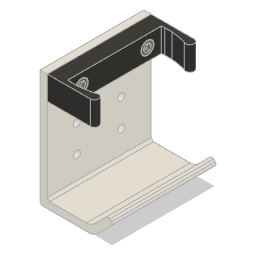
Zippo carry v8 (Autodesk Fusion 360 design; units mm, degrees)
Autodesk Fusion 360 part; units mm, degrees
note: some values were not read from the file. Chosen so that the rebuilt part matches the saved one: which bodies a step acts on. Set by a fixed rule: which sketch regions a step uses.
sketch "Sketch1" plane through (0, 0, 0) normal (1, 0, 0) x (0, 0, -1)
  line L0 (19.25, 28.375) -> (-19.25, 28.375)
  line L1 (-19.25, 28.375) -> (-19.25, -28.375)
  line L2 (-19.25, -28.375) -> (19.25, -28.375)
  line L3 (19.25, -28.375) -> (19.25, 28.375)
  line L4 (19.25, 28.375) -> (-19.25, -28.375) construction
  line L5 (-19.25, 28.375) -> (19.25, -28.375) construction
  dimension "d1" = 38.5
  dimension "d2" = 56.75
  constraint horizontal L0
  constraint perpendicular L0 L1
  constraint parallel L0 L2
  constraint parallel L1 L3
  constraint coincident L4 origin
  constraint coincident L5 origin
  measures "d1" distance of L1.end L2.end
  measures "d2" distance of L0.end L1.end
extrude "Extrude1" add sketch "Sketch1" along normal blind 14.75 makes body 1
sketch "Sketch2" plane through (0, 28.375, 0) normal (0, 1, 0) x (-1, 0, 0)
  line L0 (0, -19.25) -> (0, 19.25)
  line L1 (0, 19.25) -> (-14.75, 19.25)
  line L2 (-14.75, 19.25) -> (-14.75, -19.25)
  line L3 (-14.75, -19.25) -> (0, -19.25)
  line L4 (-7.375, 0) -> (-7.375, 19.3)
  line L5 (-14.75, 0) -> (-14.75, 18.2)
  line L6 (0, 0) -> (0, 18.2)
  spline S0 degree 5 poles (-14.75, 18.2) (-14.455, 18.2834) (-13.865, 18.443) (-12.98, 18.6605) (-11.8, 18.9061) (-10.325, 19.134) (-8.85, 19.2757) (-7.375, 19.3242) (-5.9, 19.2757) (-4.425, 19.134) (-2.95, 18.9061) (-1.77, 18.6605) (-0.885, 18.443) (-0.295, 18.2834) (0, 18.2) knots 0 0 0 0 0 0 0.1 0.2 0.3 0.4 0.5 0.6 0.7 0.8 0.9 1 1 1 1 1 1
  line L7 (-7.375, 0) -> (-7.375, -19.3)
  line L8 (-14.75, 0) -> (-14.75, -18.2)
  line L9 (0, 0) -> (0, -18.2)
  spline S1 degree 5 poles (-14.75, -18.2) (-14.455, -18.2834) (-13.865, -18.443) (-12.98, -18.6605) (-11.8, -18.9061) (-10.325, -19.134) (-8.85, -19.2757) (-7.375, -19.3242) (-5.9, -19.2757) (-4.425, -19.134) (-2.95, -18.9061) (-1.77, -18.6605) (-0.885, -18.443) (-0.295, -18.2834) (0, -18.2) knots 0 0 0 0 0 0 0.1 0.2 0.3 0.4 0.5 0.6 0.7 0.8 0.9 1 1 1 1 1 1
  dimension "d5" = 19.3
  dimension "d6" = 18.2
  dimension "d7" = 18.2
  dimension "d8" = 19.3
  dimension "d9" = 18.2
  dimension "d10" = 18.2
  constraint perpendicular L3 L4
  constraint midpoint L2 L5.start
  constraint parallel L2 L5
  constraint coincident L6.start L9.start
  constraint perpendicular L3 L6
  constraint parallel L4 L7
  constraint parallel L2 L8
  constraint parallel L0 L9
  measures "d5" distance of L4.start L4.end
  measures "d6" distance of L5.start L5.end
  measures "d7" distance of L6.start L6.end
  measures "d8" distance of L4.start L7.end
  measures "d9" distance of L5.start L8.end
  measures "d10" distance of L6.start L9.end
extrude "Extrude2" cut sketch "Sketch2" against normal blind 57 contours L0 L3 S1 | L3 L7 S1 | L3 L7 S1 | L0 L1 S0 | L2 L3 S1 | L1 L4 S0 | L1 L4 S0 | L1 L2 S0 bodies 1
extrude "Extrude3" add sketch "Sketch2" against normal blind 56.75 contours L3 L7 S1 | L3 L7 S1 | L1 L4 S0 | L1 L4 S0 bodies 1
ref_plane "WorkPlane1" through (-1, 0, 0) normal (-1, 0, 0) x (0, 0, 1)
sketch "Sketch3" plane through (0, 28.375, 0) normal (0, 1, 0) x (-1, 0, 0)
  spline S0 degree 5 poles (-8.887, 19.25) (-9.1746, 19.2311) (-9.7572, 19.1839) (-10.6348, 19.0861) (-11.8074, 18.9046) (-12.98, 18.6605) (-13.865, 18.443) (-14.455, 18.2834) (-14.75, 18.2) knots -0.397489 -0.397489 -0.397489 -0.397489 -0.397489 -0.397489 -0.3 -0.2 -0.1 0 0 0 0 0 0
  line L0 (-14.75, 18.2) -> (-14.75, -18.2)
  spline S1 degree 5 poles (-14.75, -18.2) (-14.455, -18.2834) (-13.865, -18.443) (-12.98, -18.6605) (-11.8074, -18.9046) (-10.6348, -19.0861) (-9.7572, -19.1839) (-9.1746, -19.2311) (-8.887, -19.25) knots 0 0 0 0 0 0 0.1 0.2 0.3 0.397489 0.397489 0.397489 0.397489 0.397489 0.397489
  spline S2 degree 5 poles (-8.887, -19.25) (-8.8796, -19.2505) (-8.5772, -19.2703) (-7.9798, -19.2997) (-7.375, -19.3099) (-6.7702, -19.2997) (-6.1728, -19.2703) (-5.8704, -19.2505) (-5.863, -19.25) knots 0.397489 0.397489 0.397489 0.397489 0.397489 0.397489 0.4 0.5 0.6 0.602511 0.602511 0.602511 0.602511 0.602511 0.602511
  spline S3 degree 5 poles (-5.863, -19.25) (-5.5754, -19.2311) (-4.9928, -19.1839) (-4.1152, -19.0861) (-2.9426, -18.9046) (-1.77, -18.6605) (-0.885, -18.443) (-0.295, -18.2834) (0, -18.2) knots 0.602511 0.602511 0.602511 0.602511 0.602511 0.602511 0.7 0.8 0.9 1 1 1 1 1 1
  line L1 (0, -18.2) -> (0, 18.2)
  spline S4 degree 5 poles (0, 18.2) (-0.295, 18.2834) (-0.885, 18.443) (-1.77, 18.6605) (-2.9426, 18.9046) (-4.1152, 19.0861) (-4.9928, 19.1839) (-5.5754, 19.2311) (-5.863, 19.25) knots -1 -1 -1 -1 -1 -1 -0.9 -0.8 -0.7 -0.602511 -0.602511 -0.602511 -0.602511 -0.602511 -0.602511
  spline S5 degree 5 poles (-8.887, 19.25) (-8.8796, 19.2505) (-8.5772, 19.2703) (-7.9798, 19.2997) (-7.375, 19.3099) (-6.7702, 19.2997) (-6.1728, 19.2703) (-5.8704, 19.2505) (-5.863, 19.25) knots 0.397489 0.397489 0.397489 0.397489 0.397489 0.397489 0.4 0.5 0.6 0.602511 0.602511 0.602511 0.602511 0.602511 0.602511
  spline S6 degree 3 poles (0.5, 18.5782) (0.3787, 18.6125) (0.2574, 18.6468) (0.1361, 18.6811) (-1.8474, 19.2421) (-3.8345, 19.6177) (-5.8302, 19.7489) knots -1.024673 -1.024673 -1.024673 -1.024673 -1 -1 -1 -0.602511 -0.602511 -0.602511 -0.602511
  spline S7 degree 3 poles (-8.9198, 19.7489) (-7.8905, 19.8166) (-6.8595, 19.8166) (-5.8302, 19.7489) knots 0.397489 0.397489 0.397489 0.397489 0.602511 0.602511 0.602511 0.602511
  spline S8 degree 3 poles (-8.9198, 19.7489) (-10.9155, 19.6177) (-12.9026, 19.2421) (-14.8861, 18.6811) (-15.0074, 18.6468) (-15.1287, 18.6125) (-15.25, 18.5782) knots -0.397489 -0.397489 -0.397489 -0.397489 0 0 0 0.024673 0.024673 0.024673 0.024673
  line L2 (-15.25, 18.5782) -> (-15.25, -18.5782)
  spline S9 degree 3 poles (-15.25, -18.5782) (-15.1287, -18.6125) (-15.0074, -18.6468) (-14.8861, -18.6811) (-12.9026, -19.2421) (-10.9155, -19.6177) (-8.9198, -19.7489) knots -0.024673 -0.024673 -0.024673 -0.024673 0 0 0 0.397489 0.397489 0.397489 0.397489
  spline S10 degree 3 poles (-8.9198, -19.7489) (-7.8905, -19.8166) (-6.8595, -19.8166) (-5.8302, -19.7489) knots 0.397489 0.397489 0.397489 0.397489 0.602511 0.602511 0.602511 0.602511
  spline S11 degree 3 poles (-5.8302, -19.7489) (-3.8345, -19.6177) (-1.8474, -19.2421) (0.1361, -18.6811) (0.2574, -18.6468) (0.3787, -18.6125) (0.5, -18.5782) knots 0.602511 0.602511 0.602511 0.602511 1 1 1 1.024673 1.024673 1.024673 1.024673
  line L3 (0.5, -18.5782) -> (0.5, 18.5782)
  line L4 (-7.375, -19.7997) -> (0.5, -19.7997)
  line L5 (0.5, -19.7997) -> (0.5, -18.5782)
  circle A0 centre (-16.125, -20.091) radius 1.7477
  line L6 (-16.125, -21.8387) -> (0.5, -21.8387)
  line L7 (0.5, -21.8387) -> (0.5, -19.7997)
  line L8 (0.5, 0) -> (-15.25, 0)
  line L9 (-16.125, 21.8387) -> (0.5, 21.8387)
  circle A1 centre (-16.125, 20.091) radius 1.7477
  line L10 (-7.375, 19.7997) -> (0.5, 19.7997)
  line L11 (0.5, 19.7997) -> (0.5, 18.5782)
  line L12 (0.5, 21.8387) -> (0.5, 19.7997)
  line L13 (0.5, -21.8387) -> (8, -21.8387)
  line L14 (8, -21.8387) -> (8, 21.8387)
  line L15 (8, 21.8387) -> (0.5, 21.8387)
  line L16 (0.5, 21.8387) -> (0.5, -21.8387)
  dimension "d16" = 0.5
  dimension "d17" = 7.5
  constraint coincident S10 L4.start
  constraint horizontal L4
  constraint perpendicular L4 L5
  constraint coincident L2.end A0
  constraint coincident A0 L6.start
  constraint tangent A0 L6
  constraint horizontal L6
  constraint midpoint L3 L8.start
  constraint midpoint L2 L8.end
  constraint perpendicular L2 L8
  constraint symmetric S11.end L8 S6.start
  constraint symmetric L4.start L8 L10.start
  constraint symmetric L4.end L8 L10.end
  constraint symmetric A0 L8 A1
  constraint symmetric L6.start L8 L9.start
  constraint symmetric L6.end L8 L9.end
  constraint horizontal L13
  constraint vertical L14
  constraint horizontal L15
  constraint vertical L16
  measures "d17" distance of L6.end L13.end
extrude "Extrude4" add sketch "Sketch3" along normal blind -2 and the other way blind 12 separate body contours L3 L5 L7 L11 L12 L13 L14 L15 L16 | S7 S8 L9 A1 L10 L12 L16 | A1 | S9 S10 L4 A0 L6 L7 L16 | A0 | S10 S11 L4 L5 L16 | S6 S7 L10 L11 L16 makes body 2
sketch "Sketch4" plane through (0, 26.375, 0) normal (0, 1, 0) x (-1, 0, 0)
  arc A0 (-15.25, -18.5782) -> (-16.125, -21.8387) centre (-16.125, -20.091) ccw
  line L0 (-16.125, -21.8387) -> (8, -21.8387)
  line L1 (8, -21.8387) -> (8, 21.8387)
  line L2 (8, 21.8387) -> (-16.125, 21.8387)
  arc A1 (-16.125, 21.8387) -> (-15.25, 18.5782) centre (-16.125, 20.091) ccw
  spline S0 degree 3 poles (-8.9198, 19.7489) (-9.9854, 19.6789) (-11.0432, 19.5395) (-13.4581, 19.085) (-14.526, 18.783) (-15.25, 18.5782) knots -0.399191 -0.399191 -0.399191 -0.399191 -0.225722 -0.225722 0 0 0 0
  spline S1 degree 3 poles (-5.8302, 19.7489) (-6.3445, 19.7827) (-6.8596, 19.7997) (-7.8904, 19.7997) (-8.4055, 19.7827) (-8.9198, 19.7489) knots -0.309258 -0.309258 -0.309258 -0.309258 -0.154629 -0.154629 0 0 0 0
  spline S2 degree 3 poles (0.5, 18.5782) (-0.224, 18.783) (-1.2919, 19.085) (-3.7068, 19.5395) (-4.7646, 19.6789) (-5.8302, 19.7489) knots -0.737232 -0.737232 -0.737232 -0.737232 -0.320365 -0.320365 0 0 0 0
  line L3 (0.5, 18.5782) -> (0.5, -18.5782)
  spline S3 degree 3 poles (-5.8302, -19.7489) (-4.7646, -19.6789) (-3.7068, -19.5395) (-1.2919, -19.085) (-0.224, -18.783) (0.5, -18.5782) knots -0.399191 -0.399191 -0.399191 -0.399191 -0.225722 -0.225722 0 0 0 0
  spline S4 degree 3 poles (-8.9198, -19.7489) (-8.4055, -19.7827) (-7.8904, -19.7997) (-6.8596, -19.7997) (-6.3445, -19.7827) (-5.8302, -19.7489) knots -0.309258 -0.309258 -0.309258 -0.309258 -0.154629 -0.154629 0 0 0 0
  spline S5 degree 3 poles (-15.25, -18.5782) (-14.526, -18.783) (-13.4581, -19.085) (-11.0432, -19.5395) (-9.9854, -19.6789) (-8.9198, -19.7489) knots -0.737232 -0.737232 -0.737232 -0.737232 -0.320365 -0.320365 0 0 0 0
sketch "Sketch5" plane through (4.8218, 26.375, 0) normal (0, 1, 0) x (-1, 0, 0)
sketch "Sketch6" plane through (-0.5, 0, 0) normal (1, 0, 0) x (0, 0, -1)
  line L0 (18.5782, 26.375) -> (-18.5782, 26.375)
  line L1 (-18.5782, 26.375) -> (-18.5782, 16.375)
  line L2 (-18.5782, 16.375) -> (18.5782, 16.375)
  line L3 (18.5782, 16.375) -> (18.5782, 26.375)
  line L4 (-16.5782, 18.375) -> (16.5782, 18.375)
  line L5 (16.5782, 18.375) -> (16.5782, 24.375)
  line L6 (16.5782, 24.375) -> (-16.5782, 24.375)
  line L7 (-16.5782, 24.375) -> (-16.5782, 18.375)
  circle A0 centre (-13.8282, 21.375) radius 2.75
  circle A1 centre (13.8282, 21.375) radius 2.75
  dimension "d22" = -2
  dimension "d23" = 5.5
  dimension "d24" = 5.5
  measures "d23" diameter of A0
  measures "d24" diameter of A1
extrude "Extrude5" cut sketch "Sketch6" against normal blind 3.5 contours A1 | A0 bodies 2
sketch "Sketch7" plane through (-4, 0, 0) normal (1, 0, 0) x (0, 0, -1)
  circle A0 centre (-13.8282, 21.375) radius 2.75
  circle A1 centre (-13.8282, 21.375) radius 1.675
  dimension "d27" = 3.35
  constraint concentric A0 A1
  measures "d27" diameter of A1
extrude "Extrude6" cut sketch "Sketch7" against normal blind 7.5 contours A1 bodies 2
sketch "Sketch8" plane through (-4, 0, 0) normal (1, 0, 0) x (0, 0, -1)
  circle A0 centre (13.8282, 21.375) radius 2.75
  circle A1 centre (13.8282, 21.375) radius 1.675
  dimension "d30" = 3.35
  constraint concentric A0 A1
  measures "d30" diameter of A1
extrude "Extrude7" cut sketch "Sketch8" against normal blind 16.5 contours A1 bodies 2
extrude "Extrude8" cut 1 faces at (-8, 21.375, -19.7269) along direction (1, 0, 0) blind 1 on bodies 2 bodies 2
ref_plane "WorkPlane2" through (0, 0, 0) normal (0, 0, 1) x (1, 0, 0)
sketch "Sketch9" plane through (0, 0, 0) normal (0, 0, 1) x (1, 0, 0)
  line L0 (-7, 26.375) -> (-7, 16.375)
  line L1 (-7, 16.375) -> (-0.5, 16.375)
  line L2 (-7.2, 26.375) -> (-7.2, 16.175)
  line L3 (-7.2, 16.175) -> (-0.5, 16.175)
  line L4 (-0.5, 16.175) -> (-0.5, -28.375)
  line L5 (-0.5, -28.375) -> (-0.5, -28.575)
  line L6 (-0.5, -28.575) -> (14.75, -28.55)
  line L7 (14.75, -28.55) -> (15.75, -28.55)
  line L8 (-7.2, 26.375) -> (-10.2, 26.375)
  line L9 (-10.2, 26.375) -> (-10.1099, -28.575)
  line L10 (-10.1099, -28.575) -> (-0.5, -28.575)
  line L11 (-10.1099, -28.575) -> (-10.1099, -31.575)
  line L12 (-10.1099, -31.575) -> (15.75, -31.5326)
  line L13 (15.75, -31.5326) -> (15.75, -28.55)
  dimension "d36" = 10
  dimension "d37" = 6.5
  dimension "d38" = 0.2
  dimension "d39" = 44.55
  dimension "d40" = 0.2
  dimension "d41" = 1
  dimension "d42" = 3
  dimension "d43" = 3
  constraint vertical L0
  constraint perpendicular L0 L1
  constraint perpendicular L3 L4
  constraint parallel L4 L5
  constraint perpendicular L5 L7
  constraint perpendicular L2 L8
  constraint perpendicular L6 L9
  constraint perpendicular L5 L10
  constraint perpendicular L10 L11
  constraint perpendicular L9 L12
  constraint perpendicular L7 L13
  measures "d36" distance of L0.start L0.end
  measures "d37" distance of L0.end L1.end
  measures "d39" distance of L3.end L4.end
  measures "d40" distance of L4.end L5.end
  measures "d41" distance of L6.end L7.end
  measures "d42" distance of L2.start L8.end
  measures "d43" distance of L9.end L11.end
extrude "Extrude9" add sketch "Sketch9" along normal mid plane 40 separate body makes body 3
sketch "Sketch10" plane through (-0.5, 0, 0) normal (1, 0, 0) x (0, 0, -1)
  circle A0 centre (-13.8282, 21.375) radius 2.75
  circle A1 centre (13.8282, 21.375) radius 2.75
  line L0 (18.5782, 26.375) -> (-18.5782, 26.375)
  line L1 (-18.5782, 26.375) -> (-18.5782, 16.375)
  line L2 (-18.5782, 16.375) -> (18.5782, 16.375)
  line L3 (18.5782, 16.375) -> (18.5782, 26.375)
  circle A2 centre (-13.8282, 21.375) radius 1.5
  circle A3 centre (13.8282, 21.375) radius 1.5
  dimension "d46" = 3
  dimension "d47" = 3
  constraint concentric A0 A2
  constraint concentric A1 A3
  measures "d46" diameter of A2
  measures "d47" diameter of A3
extrude "Extrude10" cut sketch "Sketch10" against normal blind 12 contours A2 | A3 bodies 3
move_body "Move1" bodies 3 to x (1, 0, 0) y (0, 1, 0) z (0, 0, 1) at (-2, 0, 0)
sketch "Sketch11" plane through (0, 0, 0) normal (0, 0, 1) x (1, 0, 0)
  line L0 (-7.1, 16.5) -> (-9.1, 16.5)
  line L1 (-9.1, 16.5) -> (-9.1, 26.5)
  line L2 (-9.1, 26.5) -> (-7.1, 26.5)
  line L3 (-7.1, 26.5) -> (-7.1, 16.5)
  spline S0 degree 5 poles (-9.1, 26.5) (-9.1881, 26.5472) (-9.3874, 26.6434) (-9.7554, 26.7926) (-10.3847, 27.0012) (-11.3643, 27.198) (-12.4122, 27.0802) (-13.3698, 26.3373) (-14.115, 24.7457) (-14.5969, 22.241) (-14.8134, 18.868) (-14.8023, 14.7586) (-14.627, 10.1019) (-14.3665, 5.1197) (-14.1031, 0.0403) (-13.9126, -4.9249) (-13.8509, -9.6096) (-13.9491, -13.9049) (-14.2209, -17.7433) (-14.6669, -21.0901) (-15.2799, -23.9334) (-15.8952, -25.8067) (-16.4225, -26.9893) (-16.8027, -27.6795) (-17, -28) knots 0 0 0 0 0 0 0.05 0.1 0.15 0.2 0.25 0.3 0.35 0.4 0.45 0.5 0.55 0.6 0.65 0.7 0.75 0.8 0.85 0.9 0.95 1 1 1 1 1 1
  spline S1 degree 3 poles (-8.1551, 28.2627) (-8.6351, 28.52) (-9.1119, 28.7036) (-9.8009, 28.8866) (-10.3178, 29.024) (-10.965, 29.1699) (-11.7999, 29.1051) (-12.5027, 29.0505) (-13.3531, 28.7883) (-14.0563, 28.2316) (-14.8349, 27.6153) (-15.3803, 26.7305) (-15.7584, 25.7133) (-16.3668, 24.0761) (-16.6309, 21.9755) (-16.7352, 19.3508) (-16.8953, 15.3166) (-16.6212, 10.0633) (-16.3468, 4.6724) (-16.1047, -0.0835) (-15.8841, -4.8798) (-15.8896, -9.0974) (-15.8958, -13.9769) (-16.2004, -18.0963) (-16.7828, -21.2014) (-17.2785, -23.8445) (-17.9797, -25.7759) (-18.7033, -26.9518) knots 0 0 0 0 0.093182 0.093182 0.093182 0.163092 0.163092 0.163092 0.221949 0.221949 0.221949 0.287118 0.287118 0.287118 0.391999 0.391999 0.391999 0.553202 0.553202 0.553202 0.695416 0.695416 0.695416 0.859946 0.859946 0.859946 1 1 1 1
  spline S2 degree 5 poles (-8.1551, 28.2627) (-8.124, 28.2359) (-8.0626, 28.1816) (-7.9731, 28.0979) (-7.8592, 27.9818) (-7.7264, 27.8285) (-7.6039, 27.6665) (-7.4927, 27.4951) (-7.3931, 27.3138) (-7.3046, 27.1232) (-7.2265, 26.9238) (-7.1715, 26.758) (-7.1342, 26.6303) (-7.1111, 26.5437) (-7.1, 26.5) knots 0 0 0 0 0 0 0.1 0.2 0.3 0.4 0.5 0.6 0.7 0.8 0.9 1 1 1 1 1 1
  spline S3 degree 5 poles (-17, -28) (-17.0737, -28.1622) (-17.2128, -28.4669) (-17.3964, -28.865) (-17.6014, -29.2827) (-17.8454, -29.6445) (-18.1374, -29.8817) (-18.5234, -30.0293) (-19.0105, -30.1149) (-19.549, -30.1511) (-20.0583, -30.1388) (-20.4502, -30.0679) (-20.6503, -29.9197) (-20.6267, -29.6677) (-20.3888, -29.2808) (-19.9672, -28.7268) (-19.5149, -28.1267) (-19.1264, -27.5785) (-18.8476, -27.1682) (-18.7033, -26.9518) knots 0 0 0 0 0 0 0.066667 0.133333 0.2 0.266667 0.333333 0.4 0.466667 0.533333 0.6 0.666667 0.733333 0.8 0.866667 0.933333 1 1 1 1 1 1
  line L4 (-19.5068, -28.1565) -> (-17.8998, -25.7471)
  line L5 (-16.5, -26.9) -> (-17.5, -29.1)
  line L6 (-15.4, -25.4) -> (-18.6, -30.6)
  point P0 (-10.5, 27)
  point P1 (-13, 26.5)
  point P2 (-14, -3)
  point P3 (-7.5, 27.5)
  point P4 (-18.5, -30)
  point P5 (-20.5, -30)
  dimension "d50" = 2
  dimension "d51" = 10
  dimension "d52" = 2
  constraint horizontal L0
  constraint vertical L1
  constraint horizontal L2
  constraint vertical L3
  constraint midpoint S1.end L4
  constraint midpoint S0.end L5
  constraint midpoint S0.end L6
  measures "d50" distance of L0.start L0.end
  measures "d51" distance of L0.start L2.end
extrude "Extrude11" add sketch "Sketch11" along normal mid plane 40 separate body makes body 4
sketch "Sketch12" plane through (-0.5, 0, 0) normal (1, 0, 0) x (0, 0, -1)
  circle A0 centre (-13.8282, 21.375) radius 2.75
  circle A1 centre (13.8282, 21.375) radius 2.75
  line L0 (18.5782, 26.375) -> (-18.5782, 26.375)
  line L1 (-18.5782, 26.375) -> (-18.5782, 16.375)
  line L2 (-18.5782, 16.375) -> (18.5782, 16.375)
  line L3 (18.5782, 16.375) -> (18.5782, 26.375)
  circle A2 centre (13.8282, 21.375) radius 1.675
  circle A3 centre (-13.8282, 21.375) radius 1.675
  dimension "d55" = 3.35
  dimension "d56" = 3.35
  constraint concentric A1 A2
  constraint concentric A0 A3
  measures "d55" diameter of A2
  measures "d56" diameter of A3
extrude "Extrude12" cut sketch "Sketch12" against normal blind 10 contours A2 | A3 bodies 4
fillet "Fillet1" radius 10.5 1 edges at (-12.1099, -31.575, 0) on bodies 3
fillet "Fillet2" radius 11 1 edges at (-12.1099, -28.575, 0) on bodies 3
fillet "Fillet3" radius 2 1 edges at (-12.2, 26.375, 0) on bodies 3
ref_plane "WorkPlane3" through (-0.5, 21.375, 0) normal (1, 0, 0) x (0, 0, 1)
split "Split1" by plane through (-0.5, 21.375, 0) normal (1, 0, 0) bodies 2 makes body 5 at (10.5833, 19.7083, 21.8387) makes body 6 at (10.5833, 19.7083, -21.8387)
move_body "Move2" bodies 6 5 to x (1, 0, 0) y (0, 1, 0) z (0, 0, 1) at (-5, 0, 0)
combine "Combine1" operation add target body 5 tool bodies 2 6
move_body "Move3" bodies 5 to x (1, 0, 0) y (0, 1, 0) z (0, 0, 1) at (0, 0, -100)
sketch "Sketch13" plane through (-7, 0, 0) normal (-1, 0, 0) x (0, 0, 1)
  circle A0 centre (-113.8282, 21.375) radius 1.675
  circle A1 centre (-86.1718, 21.375) radius 1.675
  line L0 (-78.1613, 26.375) -> (-121.8387, 26.375)
  line L1 (-121.8387, 26.375) -> (-121.8387, 16.375)
  line L2 (-121.8387, 16.375) -> (-78.1613, 16.375)
  line L3 (-78.1613, 16.375) -> (-78.1613, 26.375)
  line L4 (-121.8387, 26.375) -> (-121.8387, -19.625)
  line L5 (-78.1613, 26.375) -> (-78.1613, -19.625)
  line L6 (-78.1613, -19.625) -> (-121.8387, -19.625)
  dimension "d66" = 46
  dimension "d67" = 46
  constraint coincident L0.end L1.start
  constraint perpendicular L0 L4
  constraint coincident L0.start L3.end
  constraint perpendicular L2 L5
  measures "d66" distance of L0.end L4.end
  measures "d67" distance of L0.start L5.end
extrude "Extrude13" add sketch "Sketch13" along normal blind 3 separate body makes body 7
sketch "Sketch14" plane through (0, 0, -121.8387) normal (0, 0, -1) x (-1, 0, 0)
  line L0 (7, 26.375) -> (7, -19.625)
  line L1 (7, -19.625) -> (10, -19.625)
  line L2 (10, -19.625) -> (10, 26.375)
  line L3 (10, 26.375) -> (7, 26.375)
  line L4 (10, -19.625) -> (-11.5, -19.625)
  line L5 (-11.5, -19.625) -> (-11.5, -22.625)
  line L6 (-11.5, -22.625) -> (10, -22.625)
  line L7 (10, -22.625) -> (10, -19.625)
  dimension "d70" = 21.5
  dimension "d71" = 3
  constraint coincident L1.end L2.start
  constraint perpendicular L2 L4
  constraint perpendicular L4 L5
  constraint perpendicular L5 L6
  measures "d70" distance of L1.end L4.end
  measures "d71" distance of L4.end L5.end
sketch "Sketch15" plane through (-10, 0, 0) normal (-1, 0, 0) x (0, 0, 1)
  circle A0 centre (-113.8282, 21.375) radius 1.675
  circle A1 centre (-86.1718, 21.375) radius 1.675
  line L0 (-78.1613, 26.375) -> (-121.8387, 26.375)
  line L1 (-121.8387, 26.375) -> (-121.8387, -19.625)
  line L2 (-121.8387, -19.625) -> (-78.1613, -19.625)
  line L3 (-78.1613, -19.625) -> (-78.1613, 26.375)
  line L4 (-121.8387, -19.625) -> (-78.1613, -19.625)
  line L5 (-121.8387, -19.625) -> (-121.8387, -22.625)
  line L6 (-121.8387, -22.625) -> (-78.1613, -22.625)
  line L7 (-78.1613, -22.625) -> (-78.1613, -19.625)
  dimension "d72" = 3
  constraint coincident L1.end L2.start
  constraint coincident L2.end L3.start
  constraint perpendicular L4 L5
  constraint perpendicular L5 L6
  constraint perpendicular L4 L7
  measures "d72" distance of L1.end L5.end
extrude "Extrude14" add sketch "Sketch15" against normal blind 21.5 contours L2 L4 L5 L6 L7 bodies 7
delete_body "RemoveBody1" bodies 3
delete_body "RemoveBody2" bodies 4
delete_body "RemoveBody3" bodies 1
sketch "Sketch16" plane through (0, 0, -121.8387) normal (0, 0, -1) x (-1, 0, 0)
  line L0 (7, 26.375) -> (7, -19.625)
  line L1 (7, -19.625) -> (-11.5, -19.625)
  line L2 (-11.5, -19.625) -> (-11.5, -22.625)
  line L3 (-11.5, -22.625) -> (10, -22.625)
  line L4 (10, -22.625) -> (10, 26.375)
  line L5 (10, 26.375) -> (7, 26.375)
  line L6 (-11.5, -19.625) -> (-18.5711, -12.5539)
  line L7 (-11.5, -19.625) -> (-1.5, -19.625) construction
  line L8 (-18.5711, -12.5539) -> (-20.6924, -14.6753)
  line L9 (-20.6924, -14.6753) -> (-12.7426, -22.625)
  line L10 (-12.7426, -22.625) -> (-11.5, -22.625)
  dimension "d75" = 135
  dimension "d76" = 10
  dimension "d77" = 3
  constraint horizontal L7
  constraint coincident L1.end L2.start
  constraint perpendicular L6 L8
  constraint perpendicular L8 L9
  constraint coincident L2.end L3.start
  constraint perpendicular L2 L10
  measures "d75" angle of L6 L7
  measures "d76" distance of L1.end L6.end
  measures "d77" distance of L6.end L8.end
extrude "Extrude15" add sketch "Sketch16" against normal blind 43.667 contours L2 L6 L8 L9 L10 bodies 7
extrude "Extrude16" add 1 faces at (14.9783, -18.9751, -78.1717) along direction (0, 0, 1) blind 0.01 on bodies 7 bodies 7
extrude "Extrude17" add 1 faces at (14.9783, -18.9751, -78.1617) along direction (0, 0, 1) blind 1 on bodies 7 bodies 7
sketch "Sketch17" plane through (-10, 0, 0) normal (-1, 0, 0) x (0, 0, 1)
  circle A0 centre (-113.8282, 21.375) radius 1.675
  circle A1 centre (-86.1718, 21.375) radius 1.675
  line L0 (-78.1613, 26.375) -> (-121.8387, 26.375)
  line L1 (-121.8387, 26.375) -> (-121.8387, -22.625)
  line L2 (-121.8387, -22.625) -> (-78.1613, -22.625)
  line L3 (-78.1613, -22.625) -> (-78.1613, 26.375)
  line L4 (-78.1613, -22.625) -> (-74, -22.625)
  line L5 (-74, -22.625) -> (-74, -10)
  line L6 (-74, -10) -> (-78.1613, -10)
  line L7 (-78.1613, -10) -> (-78.1613, -22.625)
  constraint horizontal L4
  constraint vertical L5
  constraint horizontal L6
  constraint vertical L7
  constraint coincident L2.end L3.start
extrude "Extrude18" cut sketch "Sketch17" against normal blind 45 contours L3 L4 L5 L6 L7 bodies 7
fillet "Fillet4" radius 5 2 edges at (12.7426, -22.625, -100) (11.5, -19.625, -100) on bodies 7
fillet "Fillet5" radius 1 2 edges at (18.5711, -12.5539, -100) (20.6924, -14.6753, -100) on bodies 7
chamfer "Chamfer1" distance 1 angle 45 2 edges at (-7, -19.625, -100) (-10, -22.625, -100) on bodies 7
sketch "Sketch18" plane through (-10, 0, 0) normal (-1, 0, 0) x (0, 0, 1)
  line L0 (-121.8387, -21.625) -> (-78.1613, -21.625)
  line L1 (-78.1613, -21.625) -> (-78.1613, 26.375)
  line L2 (-78.1613, 26.375) -> (-121.8387, 26.375)
  line L3 (-121.8387, 26.375) -> (-121.8387, -21.625)
  circle A0 centre (-86.1718, 21.375) radius 1.675
  circle A1 centre (-113.8282, 21.375) radius 1.675
  line L4 (-90.6613, -9.125) -> (-90.6613, 13.875)
  line L5 (-90.6613, 13.875) -> (-109.3387, 13.875)
  line L6 (-109.3387, 13.875) -> (-109.3387, -9.125)
  line L7 (-109.3387, -9.125) -> (-90.6613, -9.125)
  circle A2 centre (-109.3387, 13.875) radius 1.5
  circle A3 centre (-90.6613, 13.875) radius 1.5
  circle A4 centre (-90.6613, -9.125) radius 1.5
  circle A5 centre (-109.3387, -9.125) radius 1.5
  circle A6 centre (-109.3387, 2.375) radius 1.5
  circle A7 centre (-90.6613, 2.375) radius 1.5
  dimension "d91" = -12.5
  dimension "d92" = 3
  dimension "d93" = 3
  dimension "d94" = 3
  dimension "d95" = 3
  dimension "d96" = 3
  dimension "d97" = 3
  constraint coincident L5.end L6.start
  constraint coincident L4.end L5.start
  constraint coincident L4.start L7.end
  constraint coincident L6.end L7.start
  constraint midpoint L6 A6.centre
  constraint midpoint L4 A7.centre
  measures "d92" diameter of A2
  measures "d93" diameter of A3
  measures "d94" diameter of A4
  measures "d95" diameter of A5
  measures "d96" diameter of A6
  measures "d97" diameter of A7
extrude "Extrude19" cut sketch "Sketch18" against normal blind 8 contours L4 L7 A4 | L4 L7 A4 | L4 A7 | L4 A7 | L6 L7 A5 | L6 L7 A5 | L4 L5 A3 | L4 L5 A3 | L6 A6 | L6 A6 | L5 L6 A2 | L5 L6 A2 bodies 7
sketch "Sketch19" plane through (-10, 0, 0) normal (-1, 0, 0) x (0, 0, 1)
  circle A0 centre (-90.6613, 13.875) radius 1.5
  circle A1 centre (-109.3387, 13.875) radius 1.5
  circle A2 centre (-90.6613, -9.125) radius 1.5
  circle A3 centre (-90.6613, 2.375) radius 1.5
  circle A4 centre (-109.3387, 2.375) radius 1.5
  circle A5 centre (-109.3387, -9.125) radius 1.5
  line L0 (-121.8387, -21.625) -> (-78.1613, -21.625)
  line L1 (-78.1613, -21.625) -> (-78.1613, 26.375)
  line L2 (-78.1613, 26.375) -> (-121.8387, 26.375)
  line L3 (-121.8387, 26.375) -> (-121.8387, -21.625)
  circle A6 centre (-86.1718, 21.375) radius 1.675
  circle A7 centre (-113.8282, 21.375) radius 1.675
  circle A8 centre (-113.8282, 21.375) radius 1.45
  circle A9 centre (-86.1718, 21.375) radius 1.45
  dimension "d100" = 2.9
  dimension "d101" = 2.9
  constraint concentric A7 A8
  constraint concentric A6 A9
  measures "d100" diameter of A8
  measures "d101" diameter of A9
extrude "Extrude20" add sketch "Sketch19" against normal blind 3 contours A6 | A7 bodies 7
sketch "Sketch20" plane through (-0.5, 0, 0) normal (1, 0, 0) x (0, 0, -1)
  line L0 (119.6258, 16.375) -> (119.6258, 26.375)
  line L1 (119.6258, 26.375) -> (80.3742, 26.375)
  line L2 (80.3742, 16.375) -> (80.3742, 26.375)
  line L3 (80.3742, 16.375) -> (119.6258, 16.375)
  circle A0 centre (113.8282, 21.375) radius 2.75
  circle A1 centre (86.1718, 21.375) radius 2.75
  circle A2 centre (86.1718, 21.375) radius 2.55
  circle A3 centre (113.8282, 21.375) radius 2.55
  dimension "d104" = -0.2
  dimension "d105" = -0.2
extrude "Extrude21" add sketch "Sketch20" against normal blind 3.3 separate body contours A2 | A3 makes body 8 at (-2.7, 23.8297, -86.8624) makes body 9 at (-2.7, 23.8297, -114.5188)
sketch "Sketch21" plane through (-3.8, 0, 0) normal (-1, 0, 0) x (0, 0, 1)
  circle A0 centre (-86.1718, 21.375) radius 2.55
  circle A1 centre (-86.1718, 21.375) radius 1.425
  dimension "d108" = 2.85
  constraint concentric A0 A1
  measures "d108" diameter of A1
extrude "Extrude22" add sketch "Sketch21" along normal blind 6.2 contours A1 bodies 8
delete_body "RemoveBody4" bodies 9
copy_body "CopyPasteBodies1" bodies 8 makes body 10
move_body "Align1" bodies 10 to x (0, 0, 1) y (0, 1, 0) z (-1, 0, 0) at (-90.0782, 0, -109.9218)
move_body "Move4" bodies 10 to x (0, 0, -1) y (0, 1, 0) z (1, 0, 0) at (113.4654, 0, -117.7282)
move_body "Move5" bodies 10 to x (1, 0, 0) y (0, 1, 0) z (0, 0, 1) at (-3.55, 0, 0)
sketch "Sketch22" plane through (-0.5, 0, 0) normal (1, 0, 0) x (0, 0, -1)
  circle A0 centre (86.1718, 21.375) radius 2.55
  line L0 (85.3058, 22.875) -> (84.4397, 21.375)
  line L1 (84.4397, 21.375) -> (85.3058, 19.875)
  line L2 (85.3058, 19.875) -> (87.0378, 19.875)
  line L3 (87.0378, 19.875) -> (87.9038, 21.375)
  line L4 (87.9038, 21.375) -> (87.0378, 22.875)
  line L5 (87.0378, 22.875) -> (85.3058, 22.875)
  point P0 (86.1718, 21.375)
  dimension "d111" = 1.5
  constraint coincident P0 A0.centre
  measures "d111" distance of P0 L5
extrude "Extrude23" cut sketch "Sketch22" against normal blind 1.5 contours L0 L1 L2 L3 L4 L5 bodies 8
sketch "Sketch23" plane through (-0.5064, 0, 0) normal (1, 0, 0) x (0, 0, -1)
  circle A0 centre (113.8218, 21.375) radius 2.55
  line L0 (112.9558, 22.875) -> (112.0898, 21.375)
  line L1 (112.0898, 21.375) -> (112.9558, 19.875)
  line L2 (112.9558, 19.875) -> (114.6878, 19.875)
  line L3 (114.6878, 19.875) -> (115.5539, 21.375)
  line L4 (115.5539, 21.375) -> (114.6878, 22.875)
  line L5 (114.6878, 22.875) -> (112.9558, 22.875)
  point P0 (113.8218, 21.375)
  dimension "d114" = 1.5
  constraint coincident P0 A0.centre
  measures "d114" distance of P0 L5
extrude "Extrude24" cut sketch "Sketch23" against normal blind 1.5 contours L0 L1 L2 L3 L4 L5 bodies 10
sketch "Sketch24" plane through (-10, 0, 0) normal (-1, 0, 0) x (0, 0, 1)
  circle A0 centre (-113.8282, 21.375) radius 1.45
  circle A1 centre (-86.1718, 21.375) radius 1.45
  circle A2 centre (-90.6613, 13.875) radius 1.5
  circle A3 centre (-109.3387, 13.875) radius 1.5
  circle A4 centre (-90.6613, -9.125) radius 1.5
  circle A5 centre (-90.6613, 2.375) radius 1.5
  circle A6 centre (-109.3387, 2.375) radius 1.5
  circle A7 centre (-109.3387, -9.125) radius 1.5
  line L0 (-121.8387, -21.625) -> (-78.1613, -21.625)
  line L1 (-78.1613, -21.625) -> (-78.1613, 26.375)
  line L2 (-78.1613, 26.375) -> (-121.8387, 26.375)
  line L3 (-121.8387, 26.375) -> (-121.8387, -21.625)
  line L4 (-109.3387, 13.875) -> (-90.6617, 13.875)
  line L5 (-109.3387, -9.125) -> (-90.6617, -9.125)
  line L6 (-90.6617, -9.125) -> (-90.6617, 2.375)
  line L7 (-90.6617, 2.375) -> (-90.6617, 13.875)
  line L8 (-109.3387, 13.875) -> (-109.3387, 2.375)
  line L9 (-109.3387, 2.375) -> (-109.3387, -9.125)
  line L10 (-109.3387, 2.375) -> (-90.6617, 2.375)
  circle A8 centre (-90.6613, 13.875) radius 1.5
  circle A9 centre (-90.6617, 2.375) radius 1.5
  circle A10 centre (-109.3387, 2.375) radius 1.5
  circle A11 centre (-109.3387, 13.875) radius 1.5
  circle A12 centre (-109.3387, -9.125) radius 1.5
  circle A13 centre (-90.6617, -9.125) radius 1.5
  dimension "d117" = 18.677
  dimension "d118" = 18.677
  dimension "d119" = 11.5
  dimension "d120" = 11.5
  dimension "d121" = 11.5
  dimension "d122" = 11.5
  dimension "d123" = 18.677
  dimension "d124" = 3
  dimension "d125" = 3
  dimension "d126" = 3
  dimension "d127" = 3
  dimension "d128" = 3
  dimension "d129" = 3
  constraint coincident A3.centre L4.start
  constraint horizontal L4
  constraint coincident A7.centre L5.start
  constraint horizontal L5
  constraint perpendicular L4 L6
  constraint perpendicular L4 L7
  constraint perpendicular L4 L8
  constraint coincident A6.centre L8.end
  constraint perpendicular L5 L9
  constraint perpendicular L6 L10
  constraint concentric A2 A8
  constraint coincident L6.end L7.start
  constraint concentric A3 A11
  constraint coincident L5.end L6.start
  measures "d117" distance of A3.centre L4.end
  measures "d118" distance of A7.centre L5.end
  measures "d119" distance of L5.end L6.end
  measures "d120" distance of L6.end L4.end
  measures "d121" distance of A3.centre A6.centre
  measures "d122" distance of A6.centre A7.centre
  measures "d123" distance of A6.centre L6.end
  measures "d124" diameter of A8
  measures "d125" diameter of A9
  measures "d126" diameter of A10
  measures "d127" diameter of A11
  measures "d128" diameter of A12
  measures "d129" diameter of A13
equation "d5 = ( 38.6 / 2 ) * 1 mm"
equation "d6 = ( 36.4 / 2 ) * 1 mm"
named bodies: "Zipop", "Clamps", "Body", "Clip", "Clamp", "Clamps (2)", "Main body", "Bolt_M3_1", "Bolt_M3_2"
